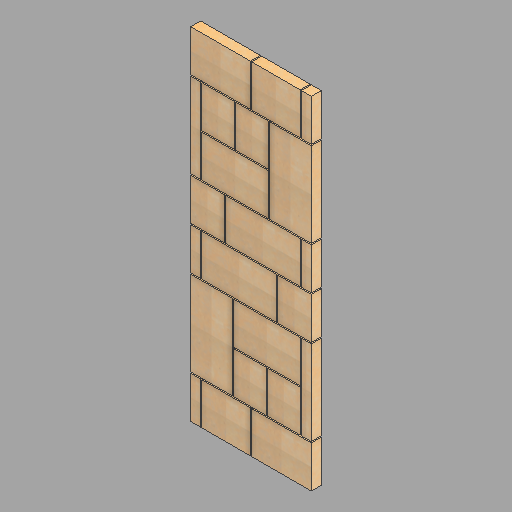
# Autodesk Inventor part: C - Split face veneer
Saved by Autodesk Inventor 2022.2 (Build 262287010, 287A)
## iProperties
RuleStatus: InUse
Created: 2022-03-23
Part Number: C - Split face veneer
Material: Granite, Cut, Polished
Document SubType Name: Modeling
Designer: awelt
Density: 2.7 g/cm^3
Appearance: Amber Select-Bolzano Edge
Mass: 1.12719e+06 g
Surface Area: 122180 cm^2
Volume: 417477 cm^3
AfterDocSave0: Convert in3 volume to ft3
in3 to ft3: 14.74
TEST: 14.743
Author: awelt
Autodesk Inventor part; units mm, degrees
ref_plane "YZ Plane" through (0, 0, 0) normal (1, 0, 0) x (0, 1, 0)
ref_plane "XZ Plane" through (0, 0, 0) normal (0, 1, 0) x (-1, 0, 0)
ref_plane "XY Plane" through (0, 0, 0) normal (0, 0, 1) x (1, 0, 0)
sketch "Sketch1" plane through (0, 0, 0) normal (0, 0, 1) x (1, 0, 0)
  line L0 (-615.95, 0) -> (615.95, 0)
  line L1 (615.95, 0) -> (615.95, 3517.9)
  line L2 (615.95, 3517.9) -> (-615.95, 3517.9)
  line L3 (-615.95, 3517.9) -> (-615.95, 0)
  line L4 (615.95, 3079.75) -> (-615.95, 3079.75)
  line L5 (615.95, 3067.05) -> (-615.95, 3067.05)
  line L6 (177.8, 2641.6) -> (-501.65, 2641.6)
  line L7 (177.8, 2628.9) -> (-501.65, 2628.9)
  line L8 (615.95, 2203.45) -> (-615.95, 2203.45)
  line L9 (615.95, 2190.75) -> (-615.95, 2190.75)
  line L10 (615.95, 1765.3) -> (-615.95, 1765.3)
  line L11 (615.95, 1752.6) -> (-615.95, 1752.6)
  line L12 (615.95, 1327.15) -> (-615.95, 1327.15)
  line L13 (615.95, 1314.45) -> (-615.95, 1314.45)
  line L14 (501.65, 889) -> (-190.5, 889)
  line L15 (501.65, 876.3) -> (-190.5, 876.3)
  line L16 (615.95, 450.85) -> (-615.95, 450.85)
  line L17 (615.95, 438.15) -> (-615.95, 438.15)
  line L18 (615.95, 3505.2) -> (-615.95, 3505.2)
  line L19 (-615.95, 12.7) -> (615.95, 12.7)
  line L20 (514.35, 1314.45) -> (514.35, 450.85)
  line L21 (514.35, 2190.75) -> (514.35, 1765.3)
  line L22 (-514.35, 1752.6) -> (-514.35, 1327.15)
  line L23 (501.65, 2190.75) -> (501.65, 1765.3)
  line L24 (-501.65, 1752.6) -> (-501.65, 1327.15)
  line L25 (501.65, 1314.45) -> (501.65, 450.85)
  line L26 (-190.5, 1314.45) -> (-190.5, 450.85)
  line L27 (-177.8, 1314.45) -> (-177.8, 450.85)
  line L28 (190.5, 3067.05) -> (190.5, 2203.45)
  line L29 (177.8, 3067.05) -> (177.8, 2203.45)
  line L30 (514.35, 3505.2) -> (514.35, 3079.75)
  line L31 (501.65, 3505.2) -> (501.65, 3079.75)
  line L32 (-514.35, 3067.05) -> (-514.35, 2203.45)
  line L33 (-501.65, 3067.05) -> (-501.65, 2203.45)
  line L34 (-514.35, 438.15) -> (-514.35, 12.7)
  line L35 (-501.65, 12.7) -> (-501.65, 438.15)
  line L36 (-6.35, 12.7) -> (-6.35, 438.15)
  line L37 (6.35, 12.7) -> (6.35, 438.15)
  line L38 (6.35, 3505.2) -> (6.35, 3079.75)
  line L39 (-6.35, 3505.2) -> (-6.35, 3079.75)
  line L40 (155.575, 876.3) -> (155.575, 450.85)
  line L41 (168.275, 876.3) -> (168.275, 450.85)
  line L42 (-155.575, 3067.05) -> (-155.575, 2641.6)
  line L43 (-168.275, 3067.05) -> (-168.275, 2641.6)
  line L44 (260.35, 1752.6) -> (260.35, 1327.15)
  line L45 (273.05, 1752.6) -> (273.05, 1327.15)
  line L46 (-260.35, 2190.75) -> (-260.35, 1765.3)
  line L47 (-273.05, 2190.75) -> (-273.05, 1765.3)
  point P0 (0, 0)
  point P1 (0, 0)
  point P2 (-177.8, 889)
  point P3 (-177.8, 876.3)
  point P4 (-177.8, 450.85)
  dimension "d0" = 3517.9
  dimension "d1" = 1231.9
  dimension "d3" = 12.7
  dimension "d4" = 425.45
  dimension "d5" = 12.7
  dimension "d6" = 425.45
  dimension "d7" = 12.7
  dimension "d8" = 425.45
  dimension "d9" = 12.7
  dimension "d10" = 425.45
  dimension "d11" = 12.7
  dimension "d12" = 425.45
  dimension "d13" = 12.7
  dimension "d14" = 425.45
  dimension "d15" = 12.7
  dimension "d16" = 12.7
  dimension "d17" = 425.45
  dimension "d18" = 12.7
  dimension "d20" = 101.6
  dimension "d21" = 101.6
  dimension "d22" = 101.6
  dimension "d25" = 425.45
  dimension "d26" = 12.7
  dimension "d27" = 12.7
  dimension "d28" = 12.7
  dimension "d30" = 425.45
  dimension "d31" = 12.7
  dimension "d32" = 425.45
  dimension "d34" = 12.7
  dimension "d35" = 101.6
  dimension "d36" = 12.7
  dimension "d37" = 101.6
  dimension "d38" = 12.7
  dimension "d39" = 101.6
  dimension "d40" = 12.7
  dimension "d46" = 609.6
  dimension "d47" = 495.3
  dimension "d48" = 495.3
  dimension "d49" = 609.6
  dimension "d50" = 333.375
  dimension "d51" = 12.7
  dimension "d52" = 333.375
  dimension "d53" = 12.7
  dimension "d55" = 762
  dimension "d56" = 12.7
  dimension "d57" = 762
  dimension "d58" = 12.7
  constraints: 96 end point, 47 point on line, 27 parallel, 16 perpendicular, 2 midpoint, 2 vertical, 1 coincident, 1 horizontal
  measures "d0" distance of L1.end L0.end
  measures "d1" distance of L0.start L0.end
  measures "d3" distance between parallel lines of L4 L5
  measures "d4" distance between parallel lines of L5 L6
  measures "d5" distance between parallel lines of L6 L7
  measures "d6" distance between parallel lines of L7 L8
  measures "d7" distance between parallel lines of L8 L9
  measures "d8" distance between parallel lines of L9 L10
  measures "d9" distance between parallel lines of L10 L11
  measures "d10" distance between parallel lines of L11 L12
  measures "d11" distance between parallel lines of L12 L13
  measures "d12" distance between parallel lines of L13 L14
  measures "d13" distance between parallel lines of L14 L15
  measures "d14" distance between parallel lines of L15 L16
  measures "d15" distance between parallel lines of L16 L17
  measures "d16" distance between parallel lines of L2 L18
  measures "d17" distance between parallel lines of L18 L4
  measures "d18" distance between parallel lines of L0 L19
  measures "d20" distance between parallel lines of L1 L20
  measures "d21" distance between parallel lines of L1 L21
  measures "d22" distance between parallel lines of L3 L22
  measures "d25" distance between parallel lines of L19 L17
  measures "d26" distance between parallel lines of L21 L23
  measures "d27" distance between parallel lines of L22 L24
  measures "d28" distance between parallel lines of L20 L25
  measures "d30" distance between parallel lines of L26 L3
  measures "d31" distance between parallel lines of L26 L27
  measures "d32" distance between parallel lines of L28 L1
  measures "d34" distance between parallel lines of L29 L28
  measures "d35" distance between parallel lines of L1 L30
  measures "d36" distance between parallel lines of L31 L30
  measures "d37" distance between parallel lines of L32 L3
  measures "d38" distance between parallel lines of L33 L32
  measures "d39" distance between parallel lines of L34 L3
  measures "d40" distance between parallel lines of L35 L34
  measures "d46" distance between parallel lines of L37 L1
  measures "d47" distance between parallel lines of L36 L35
  measures "d48" distance between parallel lines of L38 L31
  measures "d49" distance between parallel lines of L39 L3
  measures "d50" distance between parallel lines of L40 L27
  measures "d51" distance between parallel lines of L40 L41
  measures "d52" distance between parallel lines of L42 L29
  measures "d53" distance between parallel lines of L42 L43
  measures "d55" distance between parallel lines of L44 L24
  measures "d56" distance between parallel lines of L44 L45
  measures "d57" distance between parallel lines of L46 L23
  measures "d58" distance between parallel lines of L46 L47
extrude "Extrusion1" add sketch "Sketch1" along normal blind 101.6 contours L3 L18 L39 L4
extrude "Extrusion2" add sketch "Sketch1" along normal blind 101.6 separate body contours L38 L18 L31 L4
extrude "Extrusion3" add sketch "Sketch1" along normal blind 101.6 separate body contours L5 L43 L6 L33
extrude "Extrusion4" add sketch "Sketch1" along normal blind 101.6 separate body contours L29 L6 L42 L5
extrude "Extrusion5" add sketch "Sketch1" along normal blind 101.6 separate body contours L8 L28 L5 L1
extrude "Extrusion6" add sketch "Sketch1" along normal blind 101.6 separate body contours L33 L7 L29 L8
extrude "Extrusion7" add sketch "Sketch1" along normal blind 101.6 separate body contours L3 L9 L47 L10
extrude "Extrusion8" add sketch "Sketch1" along normal blind 101.6 separate body contours L46 L9 L23 L10
extrude "Extrusion9" add sketch "Sketch1" along normal blind 101.6 separate body contours L3 L13 L26 L16
extrude "Extrusion10" add sketch "Sketch1" along normal blind 101.6 separate body contours L13 L25 L14 L27
extrude "Extrusion11" add sketch "Sketch1" along normal blind 101.6 separate body contours L27 L15 L40 L16
extrude "Extrusion12" add sketch "Sketch1" along normal blind 101.6 separate body contours L16 L41 L15 L25
extrude "Extrusion13" add sketch "Sketch1" along normal blind 101.6 separate body contours L4 L30 L18 L1
extrude "Extrusion14" add sketch "Sketch1" along normal blind 101.6 separate body contours L3 L5 L32 L8
extrude "Extrusion15" add sketch "Sketch1" along normal blind 101.6 separate body contours L10 L21 L9 L1
extrude "Extrusion16" add sketch "Sketch1" along normal blind 101.6 separate body contours L3 L11 L22 L12
extrude "Extrusion17" add sketch "Sketch1" along normal blind 101.6 separate body contours L24 L11 L44 L12
extrude "Extrusion18" add sketch "Sketch1" along normal blind 101.6 separate body contours L12 L45 L11 L1
extrude "Extrusion19" add sketch "Sketch1" along normal blind 101.6 separate body contours L16 L20 L13 L1
extrude "Extrusion20" add sketch "Sketch1" along normal blind 101.6 separate body contours L3 L17 L34 L19
extrude "Extrusion21" add sketch "Sketch1" along normal blind 101.6 separate body contours L35 L17 L36 L19
extrude "Extrusion22" add sketch "Sketch1" along normal blind 101.6 separate body contours L19 L37 L17 L1
equation "\"d3\" = Joint"
equation "\"d4\" = Course"
equation "\"d5\" = Joint"
equation "\"d6\" = Course"
equation "\"d7\" = Joint"
equation "\"d8\" = Course"
equation "\"d9\" = Joint"
equation "\"d10\" = Course"
equation "\"d11\" = Joint"
equation "\"d12\" = Course"
equation "\"d13\" = Joint"
equation "\"d14\" = Course"
equation "\"d15\" = Joint"
equation "\"d17\" = Course"
equation "\"d18\" = Joint"
equation "\"d20\" = d19"
equation "\"d21\" = d19"
equation "\"d22\" = Thick"
equation "\"d26\" = Joint"
equation "\"d27\" = Joint"
equation "\"d28\" = Joint"
equation "\"d30\" = Course"
equation "\"d31\" = Joint"
equation "\"d32\" = Course"
equation "\"d34\" = Joint"
equation "\"d35\" = Thick"
equation "\"d36\" = Joint"
equation "\"d37\" = Thick"
equation "\"d38\" = Joint"
equation "\"d39\" = Thick"
equation "\"d40\" = Joint"
equation "\"d19\" = Thick"
equation "\"Thick\" = 101.6"
equation "\"Joint\" = 12.7"
equation "\"Course\" = 425.45"
